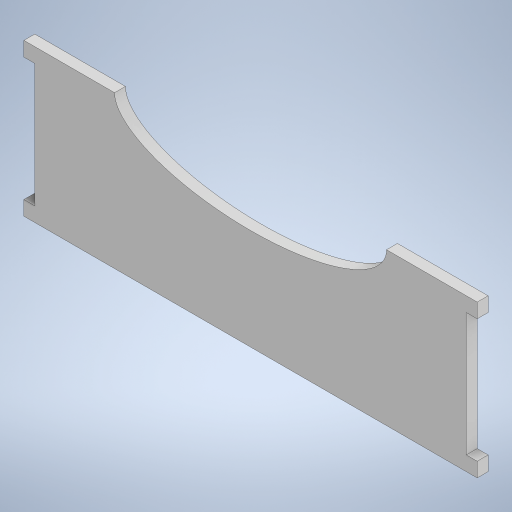
# Autodesk Inventor part: боковая стенка
Saved by Autodesk Inventor 2024.2 (Build 282272000, 272)
## iProperties
Created: 2025-11-20
Part Number: боковая стенка
Material: Типовые
Document SubType Name: Modeling
Designer: Zakhar
Density: 1 g/cm^3
Appearance: По умолчанию
Author: Zakhar
Autodesk Inventor part; units mm, degrees
ref_plane "YZ Plane" through (0, 0, 0) normal (1, 0, 0) x (0, 1, 0)
ref_plane "XZ Plane" through (0, 0, 0) normal (0, 1, 0) x (-1, 0, 0)
ref_plane "XY Plane" through (0, 0, 0) normal (0, 0, 1) x (1, 0, 0)
sketch "Эскиз1" plane through (0, 0, 0) normal (0, 0, 1) x (1, 0, 0)
  line L0 (250, 84) -> (250, 0)
  line L1 (250, 0) -> (0, 0)
  line L2 (0, 0) -> (0, 84)
  line L3 (6, 0) -> (0, 0)
  line L4 (0, 76) -> (6, 76)
  line L5 (6, 76) -> (6, 8)
  line L6 (6, 8) -> (0, 8)
  line L7 (0, 8) -> (0, 76)
  ellipse E0 centre (125, 84) end of major axis (200, 84) minor radius 28.3094 (50, 84) -> (200, 84) ccw
  line L8 (0, 84) -> (50, 84)
  line L9 (200, 84) -> (250, 84)
  line L10 (250, 76) -> (244, 76)
  line L11 (244, 76) -> (244, 8)
  line L12 (244, 8) -> (250, 8)
  line L13 (250, 8) -> (250, 76)
  point P0 (247, 8)
  point P1 (250, 8)
  point P2 (3, 76)
  point P3 (3, 0)
  point P4 (247, 76)
  dimension "d1" = 75
  dimension "d0" = 250
  dimension "d2" = 125
  dimension "d3" = 84
  dimension "d4" = 150
  dimension "d5" = 84
  dimension "d6" = 6
  dimension "d7" = 8
  dimension "d10" = 6
  dimension "d11" = 8
  dimension "d12" = 8
  dimension "d13" = 8
  dimension "d14" = 84
  constraints: 28 end point, 7 parallel, 4 horizontal, 4 midpoint, 4 perpendicular, 2 collinear, 1 coincident, 1 point on line, 4 other
  measures "d0" distance of L1.start L1.end
  measures "d2" distance of L0.start point (125, 84)
  measures "d3" distance between parallel lines of L1 L9
  measures "d4" distance of L8.end L9.start
  measures "d5" distance from line of L1 point (125, 84)
  measures "d6" distance of L13.end L11.start
  measures "d7" vertical distance of point (247, 8) L1.start
  measures "d10" distance between parallel lines of L2 L5
  measures "d11" distance from line of L8 point (3, 76)
  measures "d12" distance from line of point (3, 0) L6
  measures "d13" distance from line of L9 point (247, 76)
  measures "d14" distance between parallel lines of L1 L8
extrude "Выдавливание1" add sketch "Эскиз1" along normal blind 6 contours L0 L10 L11 L12 L1 L2 L6 L5 L4 L8 E0 L9
